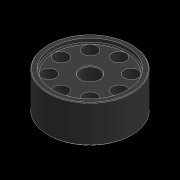
# Autodesk Inventor part: MockupWheel
Saved by Autodesk Inventor 2021 (Build 250183000, 183)
## iProperties
Created: 2021-01-23
Part Number: MockupWheel
Material: Rubber, Silicone
Document SubType Name: Modeling
Designer: Esketitttttt
Density: 1.25 g/cm^3
Appearance: Rubber - Black
Mass: 3459.55 g
Surface Area: 2382.16 cm^2
Volume: 2767.64 cm^3
Author: Esketitttttt
Autodesk Inventor part; units mm, degrees
ref_plane "YZ Plane" through (0, 0, 0) normal (1, 0, 0) x (0, 1, 0)
ref_plane "XZ Plane" through (0, 0, 0) normal (0, 1, 0) x (-1, 0, 0)
ref_plane "XY Plane" through (0, 0, 0) normal (0, 0, 1) x (1, 0, 0)
sketch "Sketch1" plane through (0, 0, 0) normal (0, 1, 0) x (-1, 0, 0)
  circle A0 centre (0, 0) radius 114.3
  circle A1 centre (0, 0) radius 12.7127
  dimension "d0" = 228.6
  dimension "d1" = 25.4254
  constraints: 2 centre point, 2 coincident
  measures "d0" diameter of A0
  measures "d1" diameter of A1
extrude "Extrusion1" add sketch "Sketch1" along normal blind 101.6
sketch "Sketch2" plane through (0, 0, 0) normal (0, -1, 0) x (1, 0, 0)
  circle A0 centre (0, 0) radius 114.3 projected
  circle A1 centre (0, 0) radius 12.7127 projected
extrude "Extrusion2" [suppressed]
sketch "Sketch3" plane through (0, 101.6, 0) normal (0, 1, 0) x (1, 0, 0)
  circle A0 centre (0, 0) radius 114.3 projected
  circle A1 centre (0, 0) radius 12.7127 projected
  circle A2 centre (0, 0) radius 101.6
  dimension "d8" = 12.7
  constraints: 1 centre point
  measures "d8" radial gap between concentric circles of A0 A2
extrude "Extrusion3" cut sketch "Sketch3" against normal blind 12.7 contours A2
fillet "Fillet1" radius 3.175 1 edges at (-101.6, 88.9, 0)
sketch "Sketch4" plane through (0, 88.9, 0) normal (0, 1, 0) x (1, 0, 0)
  circle A0 centre (0, 0) radius 12.7127 projected
  circle A1 centre (0, 0) radius 25.4
  dimension "d13" = 50.8
  constraints: 1 centre point, 1 coincident
  measures "d13" diameter of A1
extrude "SpaceForScrewSpacer" cut sketch "Sketch4" against normal through all
sketch "Sketch5" plane through (0, 63.5, 0) normal (0, 1, 0) x (1, 0, 0)
  circle A0 centre (0, 0) radius 12.7127 projected
  circle A1 centre (0, 0) radius 12.7127 projected
  line L0 (3.175, -12.3098) -> (3.175, -15.4848)
  line L1 (3.175, -15.4848) -> (-3.175, -15.4848)
  line L2 (-3.175, -12.3098) -> (-3.175, -15.4848)
  point P0 (0, -12.7127)
  dimension "d19" = 3.175
  constraints: 6 end point, 3 point on circle
  measures "d19" distance of L0.start L0.end
extrude "Keying" [suppressed]
fillet "Fillet2" radius 1.5875 3 edges at (114.3, 101.6, 0) (114.3, 0, 0) (-25.4, 88.9, 0)
sketch "Sketch6" plane through (0, 88.9, 0) normal (0, 1, 0) x (1, 0, 0)
  circle A0 centre (0, 0) radius 101.6 projected
  circle A1 centre (0, 0) radius 98.425 projected
  circle A2 centre (0, 0) radius 79.375 construction
  circle A3 centre (0, 0) radius 26.9875 projected
  circle A4 centre (79.375, 0) radius 19.05
  circle A5 centre (56.1266, 56.1266) radius 19.05
  circle A6 centre (0, 79.375) radius 19.05
  circle A7 centre (-56.1266, 56.1266) radius 19.05
  circle A8 centre (-79.375, 0) radius 19.05
  circle A9 centre (-56.1266, -56.1266) radius 19.05
  circle A10 centre (0, -79.375) radius 19.05
  circle A11 centre (56.1266, -56.1266) radius 19.05
  dimension "d23" = 158.75
  dimension "d22" = 196.85
  dimension "d24" = 53.975
  dimension "d25" = 38.1
  dimension "d28" = 360
  constraints: 8 centre point, 1 coincident, 1 horizontal alignment, 19 other
  measures "d22" diameter of A1
  measures "d24" diameter of A3
  measures "d25" diameter of A4
extrude "PocketingHoles" cut sketch "Sketch6" against normal through all contours A5 | A6 | A7 | A8 | A9 | A10 | A11 | A4
body "Solid1"
